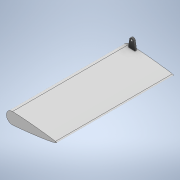
# Autodesk Inventor part: Rudder
Saved by Autodesk Inventor 2020.4 (Build 244396000, 396)
## iProperties
Created: 2021-04-29
Part Number: Rudder
Material: Generic
Document SubType Name: Modeling
Designer: armin
Density: 1 g/cm^3
Appearance: Default
Author: armin
Autodesk Inventor part; units mm, degrees
ref_plane "YZ Plane" through (0, 0, 0) normal (1, 0, 0) x (0, 1, 0)
ref_plane "XZ Plane" through (0, 0, 0) normal (0, 1, 0) x (-1, 0, 0)
ref_plane "XY Plane" through (0, 0, 0) normal (0, 0, 1) x (1, 0, 0)
sketch "Sketch21" plane through (0, 0, 0) normal (0, 0, 1) x (1, 0, 0)
  spline S0 degree 3 poles (825.3296, 54.5625) (825.7675, 54.4929) (826.1522, 54.4054) (826.4894, 54.2608) (826.573, 54.218) (826.6732, 54.1375) (826.7057, 54.1042) (826.7423, 54.0402) (826.7519, 54.0126) (826.7575, 53.9561) (826.7541, 53.9291) (826.7351, 53.868) (826.7163, 53.8353) (826.6521, 53.7491) (826.5936, 53.6974) (826.3847, 53.5396) (826.1741, 53.4325) (825.167, 52.9873) (823.8975, 52.6416) (819.2996, 51.5136) (814.2065, 50.6625) (803.9445, 49.0858) (796.6839, 48.1774) (783.2242, 46.7147) (776.0999, 46.0612) (763.0887, 45.1319) (757.1814, 44.8103) (747.9406, 44.564) (744.7861, 44.5327) (741.8194, 44.5689) knots 0 0 0 0 0.133613 0.133613 0.173725 0.173725 0.195464 0.195464 0.210211 0.210211 0.22398 0.22398 0.24206 0.24206 0.276323 0.276323 0.367098 0.367098 0.721487 0.721487 1.927938 1.927938 4.059392 4.059392 6.217603 6.217603 8.097322 8.097322 9.127359 9.127359 9.127359 9.127359
  spline S1 degree 3 poles (747.4443, 59.7341) (748.3542, 59.7869) (749.2656, 59.8329) (751.1819, 59.9164) (752.1895, 59.9527) (754.5109, 60.0208) (755.8283, 60.0478) (759.9945, 60.1011) (762.8646, 60.0898) (779.1838, 59.8066) (793.4756, 58.7082) (813.1524, 56.3704) (819.406, 55.503) (825.3296, 54.5625) knots -7.716812 -7.716812 -7.716812 -7.716812 -7.441437 -7.441437 -7.137155 -7.137155 -6.739734 -6.739734 -5.878364 -5.878364 -1.807194 -1.807194 0 0 0 0
  line L0 (774.5176, 59.7724) -> (774.2795, 45.9567)
  circle A0 centre (774.3986, 52.8646) radius 6.9066
  line L1 (829.1343, 37.5804) -> (774.4908, 37.5804)
  line L2 (774.4908, 37.5804) -> (774.4908, 70.116)
  line L3 (774.4908, 70.116) -> (829.1343, 70.116)
  line L4 (829.1343, 70.116) -> (829.1343, 37.5804)
  circle A1 centre (774.3986, 52.8646) radius 7.9066
  point P0 (0, 0)
  point P1 (719.6145, 49.2906)
  point P2 (774.3034, 45.9587)
  point P3 (774.6981, 59.7646)
  dimension "d7" = 1
  constraints: 10 end point, 2 centre point, 2 parallel, 1 coincident, 1 horizontal, 1 midpoint, 1 perpendicular, 7 other
  measures "d7" radial gap between concentric circles of A0 A1
extrude "Extrusion2" add sketch "Sketch21" along normal blind 138 contours S0 A1 S1 | S0 A0 S1 A1 | S0 L2 L0 A0 | S0 A0 L0 L2 | L0 L2 A0 | L2 L0 A0
ref_plane "Work Plane2" through (0, 0, 3.7) normal (0, 0, -1) x (-1, 0, 0)
sketch "Sketch22" plane through (0, 0, 3.7) normal (0, 0, -1) x (-1, 0, 0)
  arc A0 (-774.3034, 45.9587) -> (-774.6981, 59.7646) centre (-774.3986, 52.8646) ccw projected
  line L0 (-774.3986, 52.8646) -> (-826.6649, 54.0283)
  line L1 (-776.1113, 52.9027) -> (-778.4891, 68.8426)
  circle A1 centre (-780.9617, 68.4737) radius 2.5
  line L2 (-780.9617, 68.4737) -> (-780.9617, 53.0107)
  line L3 (-785.8122, 52.9027) -> (-783.4344, 68.8426)
  point P0 (0, 0)
  point P1 (-785.7801, 53.118)
  dimension "d11" = 5
  constraints: 8 end point, 2 point on line, 2 symmetric about line, 1 vertical, 5 other
extrude "Extrusion3" add sketch "Sketch22" along normal blind 2
sketch "Sketch23" plane through (0, 0, 3.7) normal (0, 0, 1) x (1, 0, 0)
  arc A0 (783.4344, 68.8426) -> (778.4891, 68.8426) centre (780.9617, 68.4737) ccw projected
  circle A1 centre (780.9617, 68.4737) radius 1
  point P0 (0, 0)
  dimension "d14" = 2
  constraints: 1 centre point, 1 coincident
  measures "d14" diameter of A1
extrude "Extrusion4" cut sketch "Sketch23" against normal blind 10
body "Solid2"
